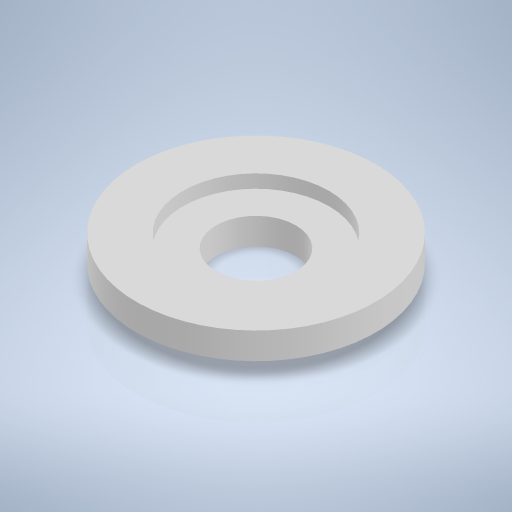
# Autodesk Inventor part: Miederhalter_ventilfeder
Saved by Autodesk Inventor 2024 (Build 280153000, 153)
## iProperties
Created: 2024-04-30
Part Number: Miederhalter_ventilfeder
Material: Generisch
Document SubType Name: Modeling
Designer: ffogue
Density: 1 g/cm^3
Appearance: Vorgabe
Author: ffogue
Autodesk Inventor part; units mm, degrees
ref_plane "YZ Plane" through (0, 0, 0) normal (1, 0, 0) x (0, 1, 0)
ref_plane "XZ Plane" through (0, 0, 0) normal (0, 1, 0) x (-1, 0, 0)
ref_plane "XY Plane" through (0, 0, 0) normal (0, 0, 1) x (1, 0, 0)
sketch "Skizze1" plane through (0, 0, 0) normal (0, 1, 0) x (-1, 0, 0)
  line L0 (0, 0) -> (4.5, 0)
  line L1 (4.5, 0) -> (4.5, -1)
  line L2 (4.5, -1) -> (3.5, -1)
  line L3 (3.5, -1) -> (3.5, -1.5)
  line L4 (3.5, -1.5) -> (0, -1.5)
  line L5 (0, -1.5) -> (0, 0)
  point P0 (4.5, -0.5)
  dimension "d0" = 1.5
  dimension "d1" = 0.5
  dimension "d2" = 9
  dimension "d3" = 7
  constraints: 12 end point, 5 perpendicular, 1 horizontal, 1 midpoint
  measures "d0" distance between parallel lines of L4 L0
  measures "d1" distance between parallel lines of L4 L2
  measures "d2" diameter of point (4.5, -0.5) L5
  measures "d3" diameter of L3 L5
revolve "Umdrehung1" add sketch "Skizze1" angle 360 about axis through (0, 0, -1.5) along (0, 0, 1)
sketch "Skizze3" plane through (0, 0, 0) normal (1, 0, 0) x (0, 1, 0)
  line L0 (0, 0) -> (2.75, 0)
  line L1 (4.5, 0) -> (-4.5, 0) projected
  line L2 (2.75, 0) -> (2.75, -0.5)
  line L3 (2.75, -0.5) -> (1.5, -0.5)
  line L4 (1.5, -0.5) -> (1.5, -1.5)
  line L5 (1.5, -1.5) -> (0, -1.5)
  line L6 (0, -1.5) -> (0, 0)
  line L7 (3.5, -1.5) -> (-3.5, -1.5) projected
  dimension "d5" = 3
  dimension "d6" = 5.5
  dimension "d7" = 0.5
  constraints: 12 end point, 4 perpendicular, 2 point on line, 1 vertical
  measures "d5" diameter of L4 L6
  measures "d6" diameter of L2 L6
  measures "d7" distance between parallel lines of L3 L0
revolve "Umdrehung2" cut sketch "Skizze3" angle 360 about axis through (0, 0, -1.5) along (0, 0, 1)
